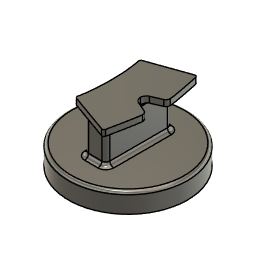
Assembly v2 (Autodesk Fusion 360 archive; units mm, degrees)
design "Joint"
Autodesk Fusion 360 part; units mm, degrees
sketch "Sketch1" plane through (0, 0, 0) normal (0, 1, 0) x (1, 0, 0)
  line L0 (8.0813, -2.7781) -> (8.0413, -2.7607)
  spline S0 degree 3 poles (-11.416, -1.3236) (-11.413, -1.5211) (-11.4109, -1.7186) (-11.4097, -1.9161) knots 0.105601 0.105601 0.105601 0.105601 0.13885 0.13885 0.13885 0.13885
  line L1 (13.1033, -27.312) -> (-13.3371, -17.9294)
  arc A0 (14.3222, -6.9462) -> (13.1249, -4.972) centre (12.3271, -6.806) ccw
  spline S1 degree 3 poles (14.3222, -6.9462) (14.3022, -7.2301) (14.2831, -7.5124) (14.2586, -7.7965) (14.2247, -8.1903) (14.1828, -8.5793) (14.129, -8.9537) (14.0945, -9.1941) (14.0671, -9.3505) (14.0481, -9.459) (13.3745, -13.3125) (12.4186, -18.2806) (11.4544, -22.7578) knots 0.129929 0.129929 0.129929 0.129929 0.210704 0.210704 0.210704 0.323115 0.323115 0.323115 0.394539 0.394539 0.394539 2.959004 2.959004 2.959004 2.959004
  line L2 (13.1441, -27.1686) -> (13.1284, -27.2237)
  spline S2 degree 3 poles (-10.7568, 0) (-10.7568, -0.0069) (-10.7568, -0.0138) (-10.757, -0.2774) (-10.7585, -0.4781) (-10.7648, -0.5732) (-10.7763, -0.6163) (-10.8404, -0.7785) (-10.9371, -0.8981) (-11.1464, -1.1124) (-11.28, -1.2227) (-11.416, -1.3236) knots -0.00207 -0.00207 -0.00207 -0.00207 0 0 0.077024 0.077024 0.142678 0.142678 0.338027 0.338027 0.559088 0.559088 0.559088 0.559088
  line L3 (6.2379, 0.0097) -> (6.2379, 0)
  line L4 (8.0833, 0) -> (-10.7568, 0)
  arc A1 (13.1249, 4.972) -> (14.3222, 6.9462) centre (12.3271, 6.806) ccw
  spline S3 degree 3 poles (-10.7568, 0) (-10.7568, 0.0069) (-10.7568, 0.0138) (-10.7569, 0.184) (-10.7584, 0.3474) (-10.7615, 0.5293) (-10.7622, 0.565) (-10.8012, 0.6906) (-10.84, 0.7582) (-11.0054, 0.9922) (-11.2011, 1.1606) (-11.3857, 1.301) (-11.4008, 1.3123) (-11.416, 1.3236) knots -0.00207 -0.00207 -0.00207 -0.00207 0 0 0.049001 0.049001 0.05468 0.05468 0.061838 0.061838 0.08267 0.08267 0.084481 0.084481 0.084481 0.084481
  line L5 (13.1284, 27.2237) -> (13.1441, 27.1686)
  line L6 (10.1423, -23.4896) -> (-9.4469, -16.5382)
  line L7 (13.1033, 27.312) -> (13.1284, 27.2237)
  line L8 (8.0813, 2.7781) -> (8.0413, 2.7607)
  spline S4 degree 3 poles (-13.3371, -17.9294) (-13.328, -17.8931) (-13.319, -17.8569) (-13.31, -17.8207) knots 0 0 0 0 0.011226 0.011226 0.011226 0.011226
  spline S5 degree 3 poles (-11.4097, 1.9161) (-11.4109, 1.7186) (-11.413, 1.5211) (-11.416, 1.3236) knots 0 0 0 0 0.059356 0.059356 0.059356 0.059356
  spline S6 degree 3 poles (17.0412, 5.8852) (17.096, 5.4635) (17.1433, 5.0656) (17.2185, 4.3576) (17.2472, 4.0451) (17.2669, 3.7791) knots -0.287448 -0.287448 -0.287448 -0.287448 -0.140551 -0.140551 0 0 0 0
  spline S7 degree 3 poles (17.2669, 3.7791) (17.2794, 3.6119) (17.2888, 3.4637) (17.3054, 3.1178) (17.3055, 2.9684) (17.2944, 2.9002) knots -0.253597 -0.253597 -0.253597 -0.253597 -0.165161 -0.165161 -0.011369 -0.011369 -0.011369 -0.011369
  spline S8 degree 3 poles (-13.31, 17.8207) (-13.319, 17.8569) (-13.328, 17.8931) (-13.3371, 17.9294) knots 0 0 0 0 0.011226 0.011226 0.011226 0.011226
  spline S9 degree 3 poles (-11.416, 1.3236) (-11.413, 1.5211) (-11.4109, 1.7186) (-11.4097, 1.9161) knots 0.105601 0.105601 0.105601 0.105601 0.13885 0.13885 0.13885 0.13885
  spline S10 degree 3 poles (13.1441, 27.1686) (13.8165, 24.2892) (14.4688, 21.1943) (15.519, 15.9244) (15.9974, 13.4078) (16.4886, 10.6628) (16.5584, 10.2683) (16.67, 9.6295) (16.7234, 9.3315) (16.868, 8.0436) (16.907, 7.4283) (16.9735, 6.5333) (17.0005, 6.1988) (17.0412, 5.8852) knots 0 0 0 0 0.887208 0.887208 1.602854 1.602854 1.722528 1.722528 1.7971 1.7971 1.874658 1.874658 1.922721 1.922721 1.922721 1.922721
  arc A2 (10.1423, -23.4896) -> (11.4544, -22.7578) centre (10.4768, -22.5472) ccw
  arc A3 (11.4544, 22.7578) -> (10.1423, 23.4896) centre (10.4768, 22.5472) ccw
  spline S11 degree 3 poles (-10.7568, 0) (-10.7568, -0.0069) (-10.7568, -0.0138) (-10.7569, -0.184) (-10.7584, -0.3474) (-10.7615, -0.5293) (-10.7622, -0.565) (-10.8012, -0.6906) (-10.84, -0.7582) (-11.0054, -0.9922) (-11.2011, -1.1606) (-11.3857, -1.301) (-11.4008, -1.3123) (-11.416, -1.3236) knots -0.00207 -0.00207 -0.00207 -0.00207 0 0 0.049001 0.049001 0.05468 0.05468 0.061838 0.061838 0.08267 0.08267 0.084481 0.084481 0.084481 0.084481
  spline S12 degree 3 poles (-10.0932, -15.4002) (-9.7612, -13.7352) (-9.4919, -12.0569) (-9.2866, -10.3718) (-9.0125, -8.1219) (-8.8527, -5.8612) (-8.8088, -3.5928) (-8.7857, -2.3952) (-8.7625, -1.1976) (-8.7394, 0) knots 0.300787 0.300787 0.300787 0.300787 0.790913 0.790913 0.790913 1.445365 1.445365 1.445365 1.804708 1.804708 1.804708 1.804708
  spline S13 degree 3 poles (14.3222, 6.9462) (14.3022, 7.2301) (14.2831, 7.5124) (14.2586, 7.7965) (14.2247, 8.1903) (14.1828, 8.5793) (14.129, 8.9537) (14.0945, 9.1941) (14.0671, 9.3505) (14.0481, 9.459) (13.3745, 13.3125) (12.4186, 18.2806) (11.4544, 22.7578) knots 0.129929 0.129929 0.129929 0.129929 0.210704 0.210704 0.210704 0.323115 0.323115 0.323115 0.394539 0.394539 0.394539 2.959004 2.959004 2.959004 2.959004
  spline S14 degree 3 poles (-10.7568, 0) (-10.7568, 0.0069) (-10.7568, 0.0138) (-10.757, 0.2774) (-10.7585, 0.4781) (-10.7648, 0.5732) (-10.7763, 0.6163) (-10.8404, 0.7785) (-10.9371, 0.8981) (-11.1464, 1.1124) (-11.28, 1.2227) (-11.416, 1.3236) knots -0.00207 -0.00207 -0.00207 -0.00207 0 0 0.077024 0.077024 0.142678 0.142678 0.338027 0.338027 0.559088 0.559088 0.559088 0.559088
  line L9 (8.0813, 2.7781) -> (13.1249, 4.972)
  spline S15 degree 3 poles (-11.4097, -1.9161) (-11.4109, -1.7186) (-11.413, -1.5211) (-11.416, -1.3236) knots 0 0 0 0 0.059356 0.059356 0.059356 0.059356
  line L10 (10.1423, 23.4896) -> (-9.4469, 16.5382)
  line L11 (13.1033, 27.312) -> (-13.3371, 17.9294)
  spline S16 degree 3 poles (17.0412, -5.8852) (16.9628, -6.4892) (16.9305, -7.2149) (16.8241, -8.4505) (16.7774, -8.8883) (16.6746, -9.603) (16.6401, -9.8004) (15.7391, -14.955) (14.387, -21.8463) (13.1441, -27.1686) knots 0 0 0 0 0.210704 0.210704 0.323115 0.323115 0.394539 0.394539 3.720426 3.720426 3.720426 3.720426
  line L12 (8.0813, -2.7781) -> (13.1249, -4.972)
  arc A4 (-10.0932, -15.4002) -> (-9.4469, -16.5382) centre (-9.1124, -15.5958) ccw
  arc A5 (-9.4469, 16.5382) -> (-10.0932, 15.4002) centre (-9.1124, 15.5958) ccw
  line L13 (13.1284, -27.2237) -> (13.1033, -27.312)
  arc A6 (6.2379, -0.0097) -> (8.0413, -2.7607) centre (9.2379, -0.0097) ccw
  arc A7 (8.0413, 2.7607) -> (6.2379, 0.0097) centre (9.2379, 0.0097) ccw
  spline S17 degree 3 poles (17.2944, -2.9002) (16.481, -2.6308) (15.6622, -2.3625) (12.7929, -1.4355) (10.7144, -0.7912) (8.6067, -0.1572) (8.4324, -0.1048) (8.258, -0.0524) (8.0833, 0) knots -0.948167 -0.948167 -0.948167 -0.948167 -0.67581 -0.67581 0 0 0 0.05588 0.05588 0.05588 0.05588
  spline S18 degree 3 poles (-11.4097, 1.9161) (-11.3936, 4.5504) (-11.5402, 7.1744) (-12.1651, 12.4904) (-12.6549, 15.1791) (-13.31, 17.8207) knots 0 0 0 0 0.791597 0.791597 1.61153 1.61153 1.61153 1.61153
  line L14 (8.0833, 0) -> (-10.7568, 0)
  spline S19 degree 3 poles (8.0833, 0) (8.2581, 0.0524) (8.4324, 0.1048) (8.6067, 0.1572) (10.8533, 0.833) (13.0674, 1.5213) (15.9303, 2.4504) (16.6142, 2.6749) (17.2944, 2.9002) knots -2.607539 -2.607539 -2.607539 -2.607539 -2.551645 -2.551645 -2.551645 -1.831287 -1.831287 -1.603516 -1.603516 -1.603516 -1.603516
  spline S20 degree 3 poles (-10.0932, 15.4002) (-9.7612, 13.7352) (-9.4919, 12.0569) (-9.2866, 10.3718) (-9.0125, 8.1219) (-8.8527, 5.8612) (-8.8088, 3.5928) (-8.7857, 2.3952) (-8.7625, 1.1976) (-8.7394, 0) knots 0.300787 0.300787 0.300787 0.300787 0.790913 0.790913 0.790913 1.445365 1.445365 1.445365 1.804708 1.804708 1.804708 1.804708
  line L15 (8.0833, 0) -> (-10.7568, 0)
  line L16 (8.0833, 0) -> (-10.7568, 0)
  spline S21 degree 3 poles (17.2669, -3.7791) (17.2472, -4.0452) (17.2185, -4.3576) (17.1433, -5.0657) (17.096, -5.4635) (17.0412, -5.8852) knots -0.28781 -0.28781 -0.28781 -0.28781 -0.147068 -0.147068 0 0 0 0
  spline S22 degree 3 poles (-13.31, -17.8207) (-12.6767, -15.2669) (-12.1979, -12.6692) (-11.5506, -7.3561) (-11.3931, -4.6416) (-11.4097, -1.9161) knots 0 0 0 0 0.790913 0.790913 1.608002 1.608002 1.608002 1.608002
  line L17 (6.2379, -0.0097) -> (6.2379, 0)
  spline S23 degree 3 poles (17.2944, -2.9002) (17.3055, -2.9682) (17.3054, -3.1169) (17.2889, -3.4621) (17.2794, -3.611) (17.2669, -3.7791) knots -0.327104 -0.327104 -0.327104 -0.327104 -0.173504 -0.173504 -0.084409 -0.084409 -0.084409 -0.084409
  dimension "d1" = 2.6121
  dimension "d2" = 3
  constraint tangent S12 A4
  constraint tangent L6 A4
  constraint tangent L6 A2
  constraint tangent S1 A2
  constraint tangent A0 L12
  constraint tangent A0 S1
  constraint coincident S12.end L4
  constraint parallel L0 L12
  constraint coincident L3.end L14
  constraint perpendicular L14 L17
  constraint tangent L0 A6
  constraint tangent A6 L17
  constraint symmetric S0.end S5.start L4
  constraint symmetric S3.end S0.start L4
  constraint symmetric L4 S5 S15
  constraint symmetric S2.start S3.start L4
  constraint symmetric S2 L4 S14
  constraint symmetric S17.end L14.start L4
  constraint symmetric L4 S3 S11
  constraint symmetric S5.start S0.end L4
  constraint symmetric S0 L4 S9
  constraint symmetric S1 L4 S13
  constraint symmetric A5.end S12.start L4
  constraint symmetric L4 A4 A5
  constraint symmetric L10.end L6.end L4
  constraint symmetric A3.start S1.end L4
  constraint symmetric L4 A2 A3
  constraint symmetric A3.end L6.start L4
  constraint symmetric L0.start L8.start L4
  constraint symmetric A1.end A0.start L4
  constraint symmetric A0 L4 A1
  constraint symmetric A0.end A1.start L4
  constraint symmetric S12.end S20.end L4
  constraint symmetric L4 S12 S20
  constraint symmetric L3.end L17.end L4
  constraint symmetric L0.end L8.end L4
  constraint symmetric A6.start L3.start L4
  constraint symmetric L4 A6 A7
  measures "d1" distance of L1 L6
  measures "d2" radius of A6
extrude "Extrude1" add sketch "Sketch1" against normal blind 3 contours L0 A0 S1 L4 L6 A2 S12 L12 A4 A6 L14 L15 L16 L17 | L3 L4 A1 L8 A3 S13 L9 L10 A5 A7 L14 S20 L15 L16
sketch "Sketch2" plane through (0, -3, 0) normal (0, -1, 0) x (1, 0, 0)
  line L0 (8.0413, 2.7607) -> (13.1249, 4.972)
  arc A0 (13.1249, 4.972) -> (14.3222, 6.9462) centre (12.3271, 6.806) ccw
  spline S0 degree 3 poles (14.3222, 6.9462) (14.3022, 7.2301) (14.2831, 7.5124) (14.2586, 7.7965) (14.2247, 8.1903) (14.1828, 8.5793) (14.129, 8.9537) (14.0945, 9.1941) (14.0671, 9.3505) (14.0481, 9.459) (13.3745, 13.3125) (12.4186, 18.2806) (11.4544, 22.7578) knots 0.129929 0.129929 0.129929 0.129929 0.210704 0.210704 0.210704 0.323115 0.323115 0.323115 0.394539 0.394539 0.394539 2.959004 2.959004 2.959004 2.959004
  arc A1 (11.4544, 22.7578) -> (10.1423, 23.4896) centre (10.4768, 22.5472) ccw
  line L1 (10.1423, 23.4896) -> (-9.4469, 16.5382)
  arc A2 (-9.4469, 16.5382) -> (-10.0932, 15.4002) centre (-9.1124, 15.5958) ccw
  spline S1 degree 3 poles (-10.0932, 15.4002) (-9.7612, 13.7352) (-9.4919, 12.0569) (-9.2866, 10.3718) (-9.0125, 8.1219) (-8.8527, 5.8612) (-8.8088, 3.5928) (-8.7857, 2.3952) (-8.7625, 1.1976) (-8.7394, 0) knots 0.300787 0.300787 0.300787 0.300787 0.790913 0.790913 0.790913 1.445365 1.445365 1.445365 1.804708 1.804708 1.804708 1.804708
  spline S2 degree 3 poles (-8.7394, 0) (-8.7625, -1.1976) (-8.7857, -2.3952) (-8.8088, -3.5928) (-8.8527, -5.8612) (-9.0125, -8.1219) (-9.2866, -10.3718) (-9.4919, -12.0569) (-9.7612, -13.7352) (-10.0932, -15.4002) knots -1.804708 -1.804708 -1.804708 -1.804708 -1.445365 -1.445365 -1.445365 -0.790913 -0.790913 -0.790913 -0.300787 -0.300787 -0.300787 -0.300787
  arc A3 (-10.0932, -15.4002) -> (-9.4469, -16.5382) centre (-9.1124, -15.5958) ccw
  line L2 (-9.4469, -16.5382) -> (10.1423, -23.4896)
  arc A4 (10.1423, -23.4896) -> (11.4544, -22.7578) centre (10.4768, -22.5472) ccw
  spline S3 degree 3 poles (11.4544, -22.7578) (12.4186, -18.2806) (13.3745, -13.3125) (14.0481, -9.459) (14.0671, -9.3505) (14.0945, -9.1941) (14.129, -8.9537) (14.1828, -8.5793) (14.2247, -8.1903) (14.2586, -7.7965) (14.2831, -7.5124) (14.3022, -7.2301) (14.3222, -6.9462) knots -2.959004 -2.959004 -2.959004 -2.959004 -0.394539 -0.394539 -0.394539 -0.323115 -0.323115 -0.323115 -0.210704 -0.210704 -0.210704 -0.129929 -0.129929 -0.129929 -0.129929
  arc A5 (14.3222, -6.9462) -> (13.1249, -4.972) centre (12.3271, -6.806) ccw
  line L3 (13.1249, -4.972) -> (8.0413, -2.7607)
  arc A6 (6.2379, -0.0097) -> (8.0413, -2.7607) centre (9.2379, -0.0097) ccw
  line L4 (6.2379, -0.0097) -> (6.2379, 0.0097)
  arc A7 (8.0413, 2.7607) -> (6.2379, 0.0097) centre (9.2379, 0.0097) ccw
  line L5 (5.3554, -16.5261) -> (-5.3554, -16.5261)
  line L6 (-5.3554, -16.5261) -> (-5.3554, 16.5261)
  line L7 (-5.3554, 16.5261) -> (5.3554, 16.5261)
  line L8 (5.3554, 16.5261) -> (5.3554, -16.5261)
  line L9 (5.3554, -16.5261) -> (-5.3554, 16.5261) construction
  line L10 (-5.3554, -16.5261) -> (5.3554, 16.5261) construction
  constraint horizontal L5
  constraint perpendicular L5 L6
  constraint parallel L5 L7
  constraint parallel L6 L8
  constraint coincident L9 origin
  constraint coincident L10 origin
extrude "Extrude2" add sketch "Sketch2" along normal blind 20 contours L5 L6 L7 L8
sketch "Sketch3" plane through (0, -23, 0) normal (0, -1, 0) x (1, 0, 0)
  line L0 (5.3554, 16.5261) -> (-5.3554, 16.5261)
  line L1 (-5.3554, 16.5261) -> (-5.3554, -16.5261)
  line L2 (-5.3554, -16.5261) -> (5.3554, -16.5261)
  line L3 (5.3554, -16.5261) -> (5.3554, 16.5261)
  circle A0 centre (0, 0) radius 30
  dimension "d7" = 60
  constraint coincident A0.centre origin
  measures "d7" diameter of A0
extrude "Extrude3" add sketch "Sketch3" along normal blind 10 contours L0 L1 L2 L3 | A0
fillet "Fillet1" radius 2 4 faces at (-5.3554, -9.6667, -5.5087) (1.7851, -9.6667, -16.5261) (5.3554, -9.6667, 5.5087) (-1.7851, -9.6667, 16.5261)
fillet "Fillet2" radius 1.5 1 edges at (-27.9698, -23, -10.8485)
